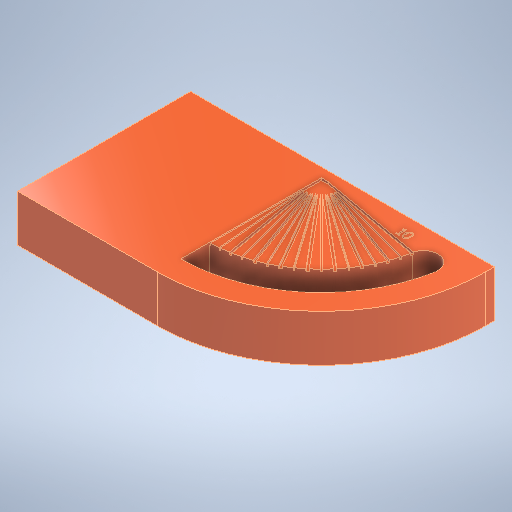
# Autodesk Inventor part: MainAnglePlate
Saved by Autodesk Inventor 2025.2 (Build 292293000, 293)
## iProperties
Created: 2025-03-13
Part Number: MainAnglePlate
Material: PET Plastic
Document SubType Name: Modeling
Designer: baolo
Density: 1.541 g/cm^3
Appearance: Smooth - Light Orange
Author: baolo
Autodesk Inventor part; units mm, degrees
ref_plane "YZ Plane" through (0, 0, 0) normal (1, 0, 0) x (0, 1, 0)
ref_plane "XZ Plane" through (0, 0, 0) normal (0, 1, 0) x (-1, 0, 0)
ref_plane "XY Plane" through (0, 0, 0) normal (0, 0, 1) x (1, 0, 0)
sketch "Sketch1" plane through (0, 0, 0) normal (0, 1, 0) x (-1, 0, 0)
  line L0 (35, 35) -> (-35, 35) construction
  line L1 (-35, 35) -> (-35, 0) construction
  line L2 (-35, 0) -> (35, 0)
  line L3 (35, 0) -> (35, 35) construction
  line L4 (35, 35) -> (-35, 0) construction
  line L5 (-35, 35) -> (35, 0) construction
  arc A0 (35, 0) -> (-35, 0) centre (0, 0) ccw
  line L6 (49, 0) -> (-49, 0) construction
  line L7 (0, -7) -> (0, 42) construction
  dimension "d0" = 70
  constraints: 12 end point, 2 midpoint, 2 parallel, 2 point on circle, 2 tangent, 1 centre point, 1 horizontal, 1 perpendicular, 1 point on line
  measures "d0" distance between parallel lines of L1 L3
extrude "Extrusion1" add sketch "Sketch1" along normal mid plane 10
sketch "Sketch3" plane through (0, 5, 0) normal (0, 1, 0) x (1, 0, 0)
  line L0 (35, 0) -> (-35, 0) construction
  arc A0 (-26.5898, -4.6885) -> (26.5898, -4.6885) centre (0, 0) ccw construction
  arc A1 (-29.5935, -5.2181) -> (29.5935, -5.2181) centre (0, 0) ccw
  arc A2 (-23.5861, -4.1589) -> (23.5861, -4.1589) centre (0, 0) ccw
  arc A3 (-23.5861, -4.1589) -> (-29.5935, -5.2181) centre (-26.5898, -4.6885) ccw
  arc A4 (29.5935, -5.2181) -> (23.5861, -4.1589) centre (26.5898, -4.6885) ccw
  arc A5 (-35, 0) -> (35, 0) centre (0, 0) ccw construction
  line L1 (-26.5898, -4.6885) -> (0, 0) construction
  line L2 (0, 0) -> (26.5898, -4.6885) construction
  dimension "d5" = 8
  dimension "d6" = 3.05
  dimension "d29" = 10
  constraints: 10 point on circle, 5 centre point, 4 end point, 4 tangent, 1 horizontal alignment, 1 midpoint
  measures "d5" radial gap between concentric circles of A5 A0
  measures "d6" radius of A3
  measures "d29" angle of L0 L2
extrude "Extrusion2" cut sketch "Sketch3" against normal through all
sketch "Sketch4" plane through (0, 5, 0) normal (0, 1, 0) x (1, 0, 0)
  line L0 (0.0434, 0.2462) -> (26.6321, -4.4421)
  line L1 (26.6321, -4.4421) -> (26.5453, -4.9345)
  line L2 (26.5453, -4.9345) -> (-0.0434, -0.2462)
  line L3 (-0.0434, -0.2462) -> (0.0434, 0.2462)
  arc A0 (-26.5018, -4.6885) -> (26.5886, -4.6885) centre (0.0434, 0.2462) ccw construction
  arc A1 (29.5935, -5.2181) -> (23.5861, -4.1589) centre (26.5898, -4.6885) ccw construction
  arc A2 (-23.5861, -4.1589) -> (-29.5935, -5.2181) centre (-26.5898, -4.6885) ccw construction
  line L4 (35, 0) -> (-35, 0) construction
  line L5 (0, 0) -> (26.5887, -4.6883) construction
  point P0 (0, 0)
  dimension "d10" = 27
  dimension "d11" = 0.5
  dimension "d23" = 10
  constraints: 11 end point, 3 midpoint, 3 perpendicular, 3 point on circle, 2 horizontal alignment, 1 centre point, 1 coincident, 1 parallel
  measures "d10" radius of A0
  measures "d11" distance between parallel lines of L2 L0
  measures "d23" angle of L4 L5
extrude "Extrusion3" cut sketch "Sketch4" against normal blind 0.5
pattern_circular "Circular Pattern1" count 19 over 180 about axis through (0, -10, 0) along (0, -1, 0) of "Extrusion3" skipped copies 18 19
sketch "Sketch5" plane through (0, 5, 0) normal (0, 1, 0) x (1, 0, 0)
  line L0 (35, 0) -> (1.4397, 0) construction
  arc A0 (-24.5564, -4.6885) -> (24.5564, -4.6885) centre (0, 0) ccw construction
  arc A1 (29.5935, -5.2181) -> (23.5861, -4.1589) centre (26.5898, -4.6885) ccw construction
  arc A2 (-23.5861, -4.1589) -> (-29.5935, -5.2181) centre (-26.5898, -4.6885) ccw construction
  line L1 (0.0324, 0.1207) -> (24.1805, -6.3497)
  line L2 (24.1805, -6.3497) -> (24.1158, -6.5912)
  line L3 (24.1158, -6.5912) -> (-0.0324, -0.1207)
  line L4 (-0.0324, -0.1207) -> (0.0324, 0.1207)
  line L5 (24.1481, -6.4705) -> (0, 0) construction
  dimension "d20" = 25
  dimension "d21" = 0.25
  dimension "d22" = 15
  constraints: 10 end point, 4 perpendicular, 3 point on circle, 2 coincident, 2 horizontal alignment, 2 midpoint, 1 centre point
  measures "d20" radius of A0
  measures "d21" distance between parallel lines of L3 L1
  measures "d22" angle of L0 L5
extrude "Extrusion4" cut sketch "Sketch5" against normal blind 0.5
pattern_circular "Circular Pattern2" count 19 over 180 about axis through (0, -10, 0) along (0, -1, 0) of "Extrusion4" skipped copies 17 18 19
sketch "Sketch6" plane through (0, 5, 0) normal (0, 1, 0) x (1, 0, 0)
  line L0 (17.9928, -0.4249) -> (37.6496, -0.4249) construction
  line L1 (37.6496, -0.4249) -> (37.6496, -4.495) construction
  line L2 (37.6496, -4.495) -> (17.9928, -4.495) construction
  line L3 (17.9928, -4.495) -> (17.9928, -0.4249) construction
  line L4 (18.8635, -2.3542) -> (18.6187, -2.3542)
  line L5 (18.6187, -2.3542) -> (18.3739, -2.3525)
  spline S0 degree 2 poles (18.3739, -2.3525) (18.2877, -2.3525) (18.2532, -2.3421) knots 0 0 0 1 1 1
  spline S1 degree 2 poles (18.2532, -2.3421) (18.1894, -2.3197) (18.1894, -2.2473) knots 0 0 0 1 1 1
  spline S2 degree 2 poles (18.1894, -2.2473) (18.1894, -2.1231) (18.3825, -2.1231) knots 0 0 0 1 1 1
  line L6 (18.3825, -2.1231) -> (18.4428, -2.1249)
  line L7 (18.4428, -2.1249) -> (18.4928, -2.1266)
  spline S3 degree 2 poles (18.4928, -2.1266) (18.4928, -2.068) (18.4721, -1.8352) (18.4721, -1.7766) knots 0 0 0 1 2 2 2
  spline S4 degree 2 poles (18.4721, -1.7766) (18.4721, -1.6197) (18.4997, -1.299) knots 0 0 0 1 1 1
  spline S5 degree 2 poles (18.4997, -1.299) (18.5273, -0.9852) (18.5256, -0.8214) knots 0 0 0 1 1 1
  spline S6 degree 2 poles (18.5256, -0.8214) (18.3601, -0.9507) (18.3152, -0.9507) knots 0 0 0 1 1 1
  spline S7 degree 2 poles (18.3152, -0.9507) (18.2652, -0.9507) (18.1928, -0.8766) (18.1928, -0.8283) knots 0 0 0 1 2 2 2
  spline S8 degree 2 poles (18.1928, -0.8283) (18.1928, -0.7697) (18.2997, -0.6869) knots 0 0 0 1 1 1
  spline S9 degree 2 poles (18.2997, -0.6869) (18.3652, -0.6387) (18.4877, -0.5352) knots 0 0 0 1 1 1
  spline S10 degree 2 poles (18.4877, -0.5352) (18.598, -0.4249) (18.6963, -0.4249) knots 0 0 0 1 1 1
  spline S11 degree 2 poles (18.6963, -0.4249) (18.779, -0.4249) (18.779, -0.5197) knots 0 0 0 1 1 1
  spline S12 degree 2 poles (18.779, -0.5197) (18.779, -0.549) (18.7635, -0.6611) (18.7635, -0.6904) knots 0 0 0 1 2 2 2
  spline S13 degree 2 poles (18.7635, -0.6904) (18.7635, -0.73) (18.7721, -0.8956) (18.7721, -0.9369) knots 0 0 0 1 2 2 2
  spline S14 degree 2 poles (18.7721, -0.9369) (18.7721, -1.0783) (18.7135, -1.6369) (18.7135, -1.7766) knots 0 0 0 1 2 2 2
  spline S15 degree 2 poles (18.7135, -1.7766) (18.7135, -1.849) (18.7325, -2.0542) (18.7342, -2.1197) knots 0 0 0 1 2 2 2
  line L8 (18.7342, -2.1197) -> (18.8635, -2.118)
  spline S16 degree 2 poles (18.8635, -2.118) (18.917, -2.118) (18.9842, -2.1852) (18.9842, -2.2352) knots 0 0 0 1 2 2 2
  spline S17 degree 2 poles (18.9842, -2.2352) (18.9842, -2.2869) (18.917, -2.3542) (18.8635, -2.3542) knots 0 0 0 1 2 2 2
  spline S18 degree 2 poles (19.8894, -2.4007) (19.5135, -2.4007) (19.3411, -2.0576) knots 0 0 0 1 1 1
  spline S19 degree 2 poles (19.3411, -2.0576) (19.2101, -1.7921) (19.2101, -1.368) knots 0 0 0 1 1 1
  spline S20 degree 2 poles (19.2101, -1.368) (19.2101, -1.0093) (19.3808, -0.7421) knots 0 0 0 1 1 1
  spline S21 degree 2 poles (19.3808, -0.7421) (19.5825, -0.43) (19.9273, -0.43) knots 0 0 0 1 1 1
  spline S22 degree 2 poles (19.9273, -0.43) (20.2532, -0.43) (20.4342, -0.7076) knots 0 0 0 1 1 1
  spline S23 degree 2 poles (20.4342, -0.7076) (20.5911, -0.9473) (20.5911, -1.2921) knots 0 0 0 1 1 1
  spline S24 degree 2 poles (20.5911, -1.2921) (20.5911, -1.8456) (20.2411, -2.4007) (19.8894, -2.4007) knots 0 0 0 1 2 2 2
  spline S25 degree 2 poles (19.9273, -0.668) (19.6963, -0.668) (19.5618, -0.9025) knots 0 0 0 1 1 1
  spline S26 degree 2 poles (19.5618, -0.9025) (19.4497, -1.0973) (19.4497, -1.3473) knots 0 0 0 1 1 1
  spline S27 degree 2 poles (19.4497, -1.3473) (19.4497, -1.7542) (19.6704, -2.1628) (19.8894, -2.1628) knots 0 0 0 1 2 2 2
  spline S28 degree 2 poles (19.8894, -2.1628) (20.1514, -2.1628) (20.2652, -1.8628) knots 0 0 0 1 1 1
  spline S29 degree 2 poles (20.2652, -1.8628) (20.3445, -1.6559) (20.3445, -1.3369) knots 0 0 0 1 1 1
  spline S30 degree 2 poles (20.3445, -1.3369) (20.3445, -1.0025) (20.1359, -0.668) (19.9273, -0.668) knots 0 0 0 1 2 2 2
  point P0 (0, 0)
  constraints: 2 other
emboss "Emboss1" sketch "Sketch6" operation cut depth 1 direction (0, -1, 0)
sketch "Sketch7" plane through (0, 5, 0) normal (0, 1, 0) x (1, 0, 0)
  line L0 (0, 0) -> (-69.9459, 0)
  line L1 (-69.9459, 0) -> (-69.9459, -63.8615)
  line L2 (-69.9459, -63.8615) -> (0, -63.8615)
  line L3 (0, -63.8615) -> (0, 0)
  constraints: 8 end point, 2 parallel, 1 horizontal, 1 perpendicular
extrude "Extrusion5" cut sketch "Sketch7" against normal through all
sketch "Sketch8" plane through (0, 0, 44.9993) normal (-1, 0, 0) x (0, 0, 1)
  line L0 (-44.9993, -5) -> (-44.9993, 4.5) construction
  line L1 (-9.9993, 5) -> (-9.9993, -5) construction
  line L2 (-44.9993, -5) -> (-44.9993, 5) projected
  line L3 (-44.9993, -5) -> (-9.9993, -5)
  line L4 (-9.9993, -5) -> (-9.9993, 5)
  line L5 (-9.9993, 5) -> (-44.9993, 5)
  line L6 (-44.9993, 5) -> (-44.9993, -5)
  point P0 (-44.9993, 5)
  constraints: 8 end point, 2 parallel, 1 horizontal, 1 perpendicular
extrude "Extrusion6" add sketch "Sketch8" along normal blind 30
sketch "Sketch10" plane through (0, -5, 0) normal (0, -1, 0) x (1, 0, 0)
  line L0 (5.7394, 2.8439) -> (-28.2134, 2.8439) construction
  line L1 (-28.2134, 2.8439) -> (-28.2134, 16.771) construction
  line L2 (-28.2134, 16.771) -> (5.7394, 16.771) construction
  line L3 (5.7394, 16.771) -> (5.7394, 2.8439) construction
  spline S0 degree 2 poles (3.3633, 4.9557) (3.3633, 5.183) (3.5362, 5.5312) (3.6794, 5.6448) knots 0 0 0 1 2 2 2
  spline S1 degree 2 poles (3.6794, 5.6448) (3.8523, 5.7782) (4.245, 5.8919) (4.5563, 5.8919) knots 0 0 0 1 2 2 2
  line L4 (4.5563, 5.8919) -> (5.4307, 5.8919)
  line L5 (5.4307, 5.8919) -> (5.4307, 2.8439)
  line L6 (5.4307, 2.8439) -> (4.623, 2.8439)
  spline S2 degree 2 poles (4.623, 2.8439) (4.2969, 2.8439) (3.9709, 2.8858) (3.8227, 2.9674) knots 0 0 0 1 2 2 2
  spline S3 degree 2 poles (3.8227, 2.9674) (3.6572, 3.0538) (3.5065, 3.3379) (3.5065, 3.5305) knots 0 0 0 1 2 2 2
  spline S4 degree 2 poles (3.5065, 3.5305) (3.5065, 3.7454) (3.7338, 4.0863) (3.9338, 4.1826) knots 0 0 0 1 2 2 2
  line L7 (3.9338, 4.1826) -> (3.9338, 4.1974)
  spline S5 degree 2 poles (3.9338, 4.1974) (3.6621, 4.2715) (3.3633, 4.6643) (3.3633, 4.9557) knots 0 0 0 1 2 2 2
  spline S6 degree 2 poles (3.7856, 4.973) (3.7856, 4.8001) (3.8844, 4.5778) (4.0326, 4.4988) knots 0 0 0 1 2 2 2
  spline S7 degree 2 poles (4.0326, 4.4988) (4.129, 4.4494) (4.3562, 4.4197) (4.5661, 4.4197) knots 0 0 0 1 2 2 2
  line L8 (4.5661, 4.4197) -> (5.0256, 4.4197)
  line L9 (5.0256, 4.4197) -> (5.0256, 5.546)
  line L10 (5.0256, 5.546) -> (4.6971, 5.546)
  spline S8 degree 2 poles (4.6971, 5.546) (4.4303, 5.546) (4.124, 5.4966) (4.0055, 5.4176) knots 0 0 0 1 2 2 2
  spline S9 degree 2 poles (4.0055, 5.4176) (3.8918, 5.3361) (3.7856, 5.1336) (3.7856, 4.973) knots 0 0 0 1 2 2 2
  spline S10 degree 2 poles (3.9289, 3.5873) (3.9289, 3.4786) (4.003, 3.3156) (4.0845, 3.2687) knots 0 0 0 1 2 2 2
  spline S11 degree 2 poles (4.0845, 3.2687) (4.1833, 3.2144) (4.4229, 3.1897) (4.6378, 3.1897) knots 0 0 0 1 2 2 2
  line L11 (4.6378, 3.1897) -> (5.0256, 3.1897)
  line L12 (5.0256, 3.1897) -> (5.0256, 4.0813)
  line L13 (5.0256, 4.0813) -> (4.5661, 4.0813)
  spline S12 degree 2 poles (4.5661, 4.0813) (4.376, 4.0813) (4.1956, 4.0418) (4.0993, 3.9801) knots 0 0 0 1 2 2 2
  spline S13 degree 2 poles (4.0993, 3.9801) (4.0055, 3.9208) (3.9289, 3.7306) (3.9289, 3.5873) knots 0 0 0 1 2 2 2
  spline S14 degree 2 poles (1.7158, 5.6498) (1.7627, 5.6844) (1.9208, 5.8079) (1.9949, 5.8449) knots 0 0 0 1 2 2 2
  spline S15 degree 2 poles (1.9949, 5.8449) (2.0961, 5.8993) (2.2863, 5.9561) (2.4592, 5.9561) knots 0 0 0 1 2 2 2
  spline S16 degree 2 poles (2.4592, 5.9561) (2.6, 5.9561) (2.8544, 5.8499) (2.9508, 5.7535) knots 0 0 0 1 2 2 2
  spline S17 degree 2 poles (2.9508, 5.7535) (3.0421, 5.6597) (3.1533, 5.383) (3.1533, 5.2299) knots 0 0 0 1 2 2 2
  spline S18 degree 2 poles (3.1533, 5.2299) (3.1533, 4.9928) (2.9532, 4.6568) (2.7359, 4.5605) knots 0 0 0 1 2 2 2
  spline S19 degree 2 poles (2.7359, 4.5605) (2.5432, 4.4716) (2.0196, 4.4049) (1.7158, 4.3876) knots 0 0 0 1 2 2 2
  line L14 (1.7158, 4.3876) -> (1.7158, 4.3135)
  spline S20 degree 2 poles (1.7158, 4.3135) (1.7158, 4.1801) (1.7973, 4.0146) (1.8714, 3.9677) knots 0 0 0 1 2 2 2
  spline S21 degree 2 poles (1.8714, 3.9677) (1.9455, 3.9208) (2.1579, 3.8911) (2.2715, 3.8911) knots 0 0 0 1 2 2 2
  spline S22 degree 2 poles (2.2715, 3.8911) (2.4049, 3.8911) (2.7655, 3.9702) (2.9458, 4.0467) knots 0 0 0 1 2 2 2
  line L15 (2.9458, 4.0467) -> (2.968, 4.0467)
  line L16 (2.968, 4.0467) -> (2.968, 3.654)
  spline S23 degree 2 poles (2.968, 3.654) (2.8618, 3.6244) (2.4642, 3.5503) (2.269, 3.5503) knots 0 0 0 1 2 2 2
  spline S24 degree 2 poles (2.269, 3.5503) (2.0319, 3.5503) (1.7083, 3.6244) (1.5799, 3.7207) knots 0 0 0 1 2 2 2
  spline S25 degree 2 poles (1.5799, 3.7207) (1.4539, 3.8146) (1.3304, 4.1134) (1.3304, 4.3283) knots 0 0 0 1 2 2 2
  line L17 (1.3304, 4.3283) -> (1.3304, 5.8919)
  line L18 (1.3304, 5.8919) -> (1.7158, 5.8919)
  line L19 (1.7158, 5.8919) -> (1.7158, 5.6498)
  line L20 (1.7158, 5.3287) -> (1.7158, 4.6939)
  spline S26 degree 2 poles (1.7158, 4.6939) (1.8541, 4.7062) (2.2715, 4.7482) (2.4024, 4.7878) knots 0 0 0 1 2 2 2
  spline S27 degree 2 poles (2.4024, 4.7878) (2.5556, 4.8347) (2.7556, 5.0298) (2.7556, 5.2027) knots 0 0 0 1 2 2 2
  spline S28 degree 2 poles (2.7556, 5.2027) (2.7556, 5.4003) (2.5333, 5.6004) (2.3209, 5.6004) knots 0 0 0 1 2 2 2
  spline S29 degree 2 poles (2.3209, 5.6004) (2.1406, 5.6004) (1.8442, 5.4448) (1.7158, 5.3287) knots 0 0 0 1 2 2 2
  spline S30 degree 2 poles (-1.0902, 4.7482) (-1.0902, 5.3262) (-0.5344, 5.9561) (-0.0701, 5.9561) knots 0 0 0 1 2 2 2
  spline S31 degree 2 poles (-0.0701, 5.9561) (0.4066, 5.9561) (0.9525, 5.3065) (0.9525, 4.7482) knots 0 0 0 1 2 2 2
  spline S32 degree 2 poles (0.9525, 4.7482) (0.9525, 4.1752) (0.3894, 3.5404) (-0.0701, 3.5404) knots 0 0 0 1 2 2 2
  spline S33 degree 2 poles (-0.0701, 3.5404) (-0.5344, 3.5404) (-1.0902, 4.1727) (-1.0902, 4.7482) knots 0 0 0 1 2 2 2
  spline S34 degree 2 poles (-0.6925, 4.7482) (-0.6925, 4.3036) (-0.3689, 3.8714) (-0.0701, 3.8714) knots 0 0 0 1 2 2 2
  spline S35 degree 2 poles (-0.0701, 3.8714) (0.2288, 3.8714) (0.5548, 4.3036) (0.5548, 4.7482) knots 0 0 0 1 2 2 2
  spline S36 degree 2 poles (0.5548, 4.7482) (0.5548, 5.1805) (0.2288, 5.6251) (-0.0701, 5.6251) knots 0 0 0 1 2 2 2
  spline S37 degree 2 poles (-0.0701, 5.6251) (-0.3665, 5.6251) (-0.6925, 5.1879) (-0.6925, 4.7482) knots 0 0 0 1 2 2 2
  line L21 (-5.0052, 5.8919) -> (-4.5507, 5.8919)
  line L22 (-4.5507, 5.8919) -> (-3.2021, 3.2638)
  line L23 (-3.2021, 3.2638) -> (-3.2021, 5.8919)
  line L24 (-3.2021, 5.8919) -> (-2.8241, 5.8919)
  line L25 (-2.8241, 5.8919) -> (-2.8241, 2.8439)
  line L26 (-2.8241, 2.8439) -> (-3.3997, 2.8439)
  line L27 (-3.3997, 2.8439) -> (-4.6273, 5.2571)
  line L28 (-4.6273, 5.2571) -> (-4.6273, 2.8439)
  line L29 (-4.6273, 2.8439) -> (-5.0052, 2.8439)
  line L30 (-5.0052, 2.8439) -> (-5.0052, 5.8919)
  line L31 (-6.1908, 5.8919) -> (-5.7017, 5.8919)
  line L32 (-5.7017, 5.8919) -> (-5.7017, 5.3089)
  line L33 (-5.7017, 5.3089) -> (-6.1908, 5.3089)
  line L34 (-6.1908, 5.3089) -> (-6.1908, 5.8919)
  line L35 (4.287, 11.7526) -> (4.7563, 11.7526)
  spline S38 degree 2 poles (4.7563, 11.7526) (5.112, 11.3302) (5.5196, 10.3842) (5.5196, 9.7395) knots 0 0 0 1 2 2 2
  spline S39 degree 2 poles (5.5196, 9.7395) (5.5196, 9.1097) (5.117, 8.1488) (4.7563, 7.7265) knots 0 0 0 1 2 2 2
  line L36 (4.7563, 7.7265) -> (4.287, 7.7265)
  line L37 (4.287, 7.7265) -> (4.287, 7.7462)
  spline S40 degree 2 poles (4.287, 7.7462) (4.4525, 7.8969) (4.7539, 8.2871) (4.8823, 8.5465) knots 0 0 0 1 2 2 2
  spline S41 degree 2 poles (4.8823, 8.5465) (5.0058, 8.7984) (5.159, 9.4036) (5.159, 9.7395) knots 0 0 0 1 2 2 2
  spline S42 degree 2 poles (5.159, 9.7395) (5.159, 10.0903) (5.0108, 10.6707) (4.8823, 10.9325) knots 0 0 0 1 2 2 2
  spline S43 degree 2 poles (4.8823, 10.9325) (4.7588, 11.1845) (4.4451, 11.592) (4.287, 11.7328) knots 0 0 0 1 2 2 2
  line L38 (4.287, 11.7328) -> (4.287, 11.7526)
  line L39 (3.8251, 10.9103) -> (3.8251, 7.8623)
  line L40 (3.8251, 7.8623) -> (1.9183, 7.8623)
  line L41 (1.9183, 7.8623) -> (1.9183, 8.2229)
  line L42 (1.9183, 8.2229) -> (3.4201, 8.2229)
  line L43 (3.4201, 8.2229) -> (3.4201, 9.0578)
  line L44 (3.4201, 9.0578) -> (2.0196, 9.0578)
  line L45 (2.0196, 9.0578) -> (2.0196, 9.4184)
  line L46 (2.0196, 9.4184) -> (3.4201, 9.4184)
  line L47 (3.4201, 9.4184) -> (3.4201, 10.5497)
  line L48 (3.4201, 10.5497) -> (1.9183, 10.5497)
  line L49 (1.9183, 10.5497) -> (1.9183, 10.9103)
  line L50 (1.9183, 10.9103) -> (3.8251, 10.9103)
  line L51 (-0.3195, 10.9103) -> (1.5601, 10.9103)
  line L52 (1.5601, 10.9103) -> (1.5601, 10.478)
  spline S44 degree 2 poles (1.5601, 10.478) (1.3576, 10.2879) (0.997, 9.9346) (0.8241, 9.7445) knots 0 0 0 1 2 2 2
  spline S45 degree 2 poles (0.8241, 9.7445) (0.4758, 9.3616) (0.2214, 8.9022) (0.2214, 8.6576) knots 0 0 0 1 2 2 2
  spline S46 degree 2 poles (0.2214, 8.6576) (0.2214, 8.5292) (0.3004, 8.3365) (0.3721, 8.2748) knots 0 0 0 1 2 2 2
  spline S47 degree 2 poles (0.3721, 8.2748) (0.4437, 8.213) (0.6314, 8.1513) (0.745, 8.1513) knots 0 0 0 1 2 2 2
  spline S48 degree 2 poles (0.745, 8.1513) (0.8537, 8.1513) (1.076, 8.2056) (1.1773, 8.2476) knots 0 0 0 1 2 2 2
  spline S49 degree 2 poles (1.1773, 8.2476) (1.2637, 8.2822) (1.4243, 8.381) (1.4737, 8.4156) knots 0 0 0 1 2 2 2
  line L53 (1.4737, 8.4156) -> (1.4959, 8.4156)
  line L54 (1.4959, 8.4156) -> (1.4959, 7.9809)
  spline S50 degree 2 poles (1.4959, 7.9809) (1.3699, 7.9191) (0.9179, 7.7981) (0.7154, 7.7981) knots 0 0 0 1 2 2 2
  spline S51 degree 2 poles (0.7154, 7.7981) (0.2881, 7.7981) (-0.1936, 8.2501) (-0.1936, 8.6354) knots 0 0 0 1 2 2 2
  spline S52 degree 2 poles (-0.1936, 8.6354) (-0.1936, 8.8157) (-0.1096, 9.1171) (-0.0355, 9.2455) knots 0 0 0 1 2 2 2
  spline S53 degree 2 poles (-0.0355, 9.2455) (0.0386, 9.3789) (0.2535, 9.6407) (0.3721, 9.7667) knots 0 0 0 1 2 2 2
  spline S54 degree 2 poles (0.3721, 9.7667) (0.5647, 9.9766) (1.0365, 10.4262) (1.1773, 10.5571) knots 0 0 0 1 2 2 2
  line L55 (1.1773, 10.5571) -> (-0.3195, 10.5571)
  line L56 (-0.3195, 10.5571) -> (-0.3195, 10.9103)
  line L57 (-1.8435, 9.7617) -> (-0.69, 9.7617)
  line L58 (-0.69, 9.7617) -> (-0.69, 9.3912)
  line L59 (-0.69, 9.3912) -> (-1.8435, 9.3912)
  line L60 (-1.8435, 9.3912) -> (-1.8435, 9.7617)
  line L61 (-3.9752, 10.9103) -> (-2.4882, 10.9103)
  line L62 (-2.4882, 10.9103) -> (-2.4882, 10.5991)
  line L63 (-2.4882, 10.5991) -> (-3.0415, 10.5991)
  line L64 (-3.0415, 10.5991) -> (-3.0415, 8.5564)
  line L65 (-3.0415, 8.5564) -> (-2.4882, 8.5564)
  line L66 (-2.4882, 8.5564) -> (-2.4882, 8.2773)
  spline S55 degree 2 poles (-2.4882, 8.2773) (-2.8019, 8.2773) (-3.0983, 8.0994) (-3.1181, 7.8524) knots 0 0 0 1 2 2 2
  line L67 (-3.1181, 7.8524) -> (-3.4342, 7.8524)
  line L68 (-3.4342, 7.8524) -> (-3.4342, 10.5991)
  line L69 (-3.4342, 10.5991) -> (-3.9752, 10.5991)
  line L70 (-3.9752, 10.5991) -> (-3.9752, 10.9103)
  spline S56 degree 2 poles (-5.3584, 8.1513) (-5.2472, 8.1513) (-5.0274, 8.2056) (-4.9212, 8.2476) knots 0 0 0 1 2 2 2
  spline S57 degree 2 poles (-4.9212, 8.2476) (-4.8224, 8.2896) (-4.6767, 8.3785) (-4.6198, 8.4181) knots 0 0 0 1 2 2 2
  line L71 (-4.6198, 8.4181) -> (-4.5951, 8.4181)
  line L72 (-4.5951, 8.4181) -> (-4.5951, 7.9858)
  spline S58 degree 2 poles (-4.5951, 7.9858) (-4.7285, 7.9142) (-5.1855, 7.7981) (-5.3905, 7.7981) knots 0 0 0 1 2 2 2
  spline S59 degree 2 poles (-5.3905, 7.7981) (-5.598, 7.7981) (-5.9067, 7.8821) (-6.0327, 7.971) knots 0 0 0 1 2 2 2
  spline S60 degree 2 poles (-6.0327, 7.971) (-6.1661, 8.0673) (-6.3044, 8.3464) (-6.3044, 8.5341) knots 0 0 0 1 2 2 2
  spline S61 degree 2 poles (-6.3044, 8.5341) (-6.3044, 8.7861) (-5.9734, 9.1665) (-5.7412, 9.2159) knots 0 0 0 1 2 2 2
  line L73 (-5.7412, 9.2159) -> (-5.7412, 9.2455)
  spline S62 degree 2 poles (-5.7412, 9.2455) (-5.8376, 9.2653) (-6.0574, 9.3542) (-6.1513, 9.4431) knots 0 0 0 1 2 2 2
  spline S63 degree 2 poles (-6.1513, 9.4431) (-6.2451, 9.5296) (-6.3637, 9.8062) (-6.3637, 10.0063) knots 0 0 0 1 2 2 2
  spline S64 degree 2 poles (-6.3637, 10.0063) (-6.3637, 10.2113) (-6.2229, 10.5596) (-6.0944, 10.6929) knots 0 0 0 1 2 2 2
  spline S65 degree 2 poles (-6.0944, 10.6929) (-5.9611, 10.8313) (-5.5831, 10.9745) (-5.3436, 10.9745) knots 0 0 0 1 2 2 2
  spline S66 degree 2 poles (-5.3436, 10.9745) (-5.1138, 10.9745) (-4.6643, 10.8634) (-4.5112, 10.7868) knots 0 0 0 1 2 2 2
  line L74 (-4.5112, 10.7868) -> (-4.5112, 10.3545)
  line L75 (-4.5112, 10.3545) -> (-4.5408, 10.3545)
  spline S67 degree 2 poles (-4.5408, 10.3545) (-4.6692, 10.4484) (-5.104, 10.6213) (-5.3189, 10.6213) knots 0 0 0 1 2 2 2
  spline S68 degree 2 poles (-5.3189, 10.6213) (-5.4448, 10.6213) (-5.6968, 10.5423) (-5.7807, 10.4509) knots 0 0 0 1 2 2 2
  spline S69 degree 2 poles (-5.7807, 10.4509) (-5.8623, 10.3595) (-5.9487, 10.1421) (-5.9487, 9.9766) knots 0 0 0 1 2 2 2
  spline S70 degree 2 poles (-5.9487, 9.9766) (-5.9487, 9.8111) (-5.8524, 9.5963) (-5.7659, 9.5345) knots 0 0 0 1 2 2 2
  spline S71 degree 2 poles (-5.7659, 9.5345) (-5.6795, 9.4728) (-5.4448, 9.4258) (-5.3065, 9.4258) knots 0 0 0 1 2 2 2
  line L76 (-5.3065, 9.4258) -> (-5.1336, 9.4258)
  line L77 (-5.1336, 9.4258) -> (-5.1336, 9.0874)
  line L78 (-5.1336, 9.0874) -> (-5.2695, 9.0874)
  spline S72 degree 2 poles (-5.2695, 9.0874) (-5.5436, 9.0874) (-5.8894, 8.8256) (-5.8894, 8.5761) knots 0 0 0 1 2 2 2
  spline S73 degree 2 poles (-5.8894, 8.5761) (-5.8894, 8.46) (-5.8005, 8.2946) (-5.7289, 8.2452) knots 0 0 0 1 2 2 2
  spline S74 degree 2 poles (-5.7289, 8.2452) (-5.6523, 8.1933) (-5.4646, 8.1513) (-5.3584, 8.1513) knots 0 0 0 1 2 2 2
  line L79 (-8.93, 10.9103) -> (-8.93, 8.2229)
  line L80 (-8.93, 8.2229) -> (-7.9074, 8.2229)
  line L81 (-7.9074, 8.2229) -> (-7.9074, 7.8623)
  line L82 (-7.9074, 7.8623) -> (-10.3577, 7.8623)
  line L83 (-10.3577, 7.8623) -> (-10.3577, 8.2229)
  line L84 (-10.3577, 8.2229) -> (-9.3351, 8.2229)
  line L85 (-9.3351, 8.2229) -> (-9.3351, 10.9103)
  line L86 (-9.3351, 10.9103) -> (-8.93, 10.9103)
  line L87 (-11.8496, 9.0356) -> (-11.8298, 9.0356)
  spline S75 degree 2 poles (-11.8298, 9.0356) (-11.7854, 9.0232) (-11.689, 9.0183) (-11.6223, 9.0183) knots 0 0 0 1 2 2 2
  spline S76 degree 2 poles (-11.6223, 9.0183) (-11.4667, 9.0183) (-11.1604, 9.1541) (-11.0221, 9.2875) knots 0 0 0 1 2 2 2
  line L88 (-11.0221, 9.2875) -> (-11.0221, 10.9103)
  line L89 (-11.0221, 10.9103) -> (-10.6368, 10.9103)
  line L90 (-10.6368, 10.9103) -> (-10.6368, 8.6231)
  line L91 (-10.6368, 8.6231) -> (-11.0221, 8.6231)
  line L92 (-11.0221, 8.6231) -> (-11.0221, 8.9639)
  spline S77 degree 2 poles (-11.0221, 8.9639) (-11.2321, 8.7762) (-11.5458, 8.6231) (-11.694, 8.6231) knots 0 0 0 1 2 2 2
  spline S78 degree 2 poles (-11.694, 8.6231) (-11.7532, 8.6231) (-11.8125, 8.628) (-11.8496, 8.6354) knots 0 0 0 1 2 2 2
  line L93 (-11.8496, 8.6354) -> (-11.8496, 9.0356)
  spline S79 degree 2 poles (-13.1414, 10.9622) (-12.5931, 10.9622) (-11.9904, 10.3471) (-11.9904, 9.779) knots 0 0 0 1 2 2 2
  spline S80 degree 2 poles (-11.9904, 9.779) (-11.9904, 9.2208) (-12.5758, 8.5588) (-13.0475, 8.5588) knots 0 0 0 1 2 2 2
  spline S81 degree 2 poles (-13.0475, 8.5588) (-13.26, 8.5588) (-13.5885, 8.6823) (-13.7095, 8.8133) knots 0 0 0 1 2 2 2
  spline S82 degree 2 poles (-13.7095, 8.8133) (-13.833, 8.9442) (-13.9639, 9.3221) (-13.9639, 9.5963) knots 0 0 0 1 2 2 2
  line L94 (-13.9639, 9.5963) -> (-13.9639, 9.8062)
  line L95 (-13.9639, 9.8062) -> (-12.3806, 9.8062)
  spline S83 degree 2 poles (-12.3806, 9.8062) (-12.3806, 10.2039) (-12.7808, 10.6263) (-13.1365, 10.6263) knots 0 0 0 1 2 2 2
  spline S84 degree 2 poles (-13.1365, 10.6263) (-13.2624, 10.6263) (-13.507, 10.5694) (-13.6058, 10.525) knots 0 0 0 1 2 2 2
  spline S85 degree 2 poles (-13.6058, 10.525) (-13.7095, 10.4756) (-13.8528, 10.3891) (-13.8997, 10.3496) knots 0 0 0 1 2 2 2
  line L96 (-13.8997, 10.3496) -> (-13.9219, 10.3496)
  line L97 (-13.9219, 10.3496) -> (-13.9219, 10.7695)
  spline S86 degree 2 poles (-13.9219, 10.7695) (-13.8552, 10.7967) (-13.6527, 10.8757) (-13.5736, 10.898) knots 0 0 0 1 2 2 2
  spline S87 degree 2 poles (-13.5736, 10.898) (-13.4625, 10.9301) (-13.2797, 10.9622) (-13.1414, 10.9622) knots 0 0 0 1 2 2 2
  spline S88 degree 2 poles (-13.5885, 9.5123) (-13.5835, 9.3567) (-13.5193, 9.1294) (-13.4576, 9.0529) knots 0 0 0 1 2 2 2
  spline S89 degree 2 poles (-13.4576, 9.0529) (-13.3909, 8.9664) (-13.1809, 8.875) (-13.0253, 8.875) knots 0 0 0 1 2 2 2
  spline S90 degree 2 poles (-13.0253, 8.875) (-12.8722, 8.875) (-12.6573, 8.9664) (-12.5684, 9.0553) knots 0 0 0 1 2 2 2
  spline S91 degree 2 poles (-12.5684, 9.0553) (-12.4819, 9.1467) (-12.393, 9.3665) (-12.3806, 9.5123) knots 0 0 0 1 2 2 2
  line L98 (-12.3806, 9.5123) -> (-13.5885, 9.5123)
  spline S92 degree 2 poles (-16.2709, 9.7296) (-16.2709, 10.2903) (-15.7275, 10.9745) (-15.3175, 10.9745) knots 0 0 0 1 2 2 2
  spline S93 degree 2 poles (-15.3175, 10.9745) (-15.1322, 10.9745) (-14.8679, 10.8831) (-14.7395, 10.8041) knots 0 0 0 1 2 2 2
  line L99 (-14.7395, 10.8041) -> (-14.7148, 10.9103)
  line L100 (-14.7148, 10.9103) -> (-14.3542, 10.9103)
  line L101 (-14.3542, 10.9103) -> (-14.3542, 7.7265)
  line L102 (-14.3542, 7.7265) -> (-14.7395, 7.7265)
  line L103 (-14.7395, 7.7265) -> (-14.7395, 8.8627)
  spline S94 degree 2 poles (-14.7395, 8.8627) (-14.8852, 8.7317) (-15.2236, 8.5588) (-15.4385, 8.5588) knots 0 0 0 1 2 2 2
  spline S95 degree 2 poles (-15.4385, 8.5588) (-15.8263, 8.5588) (-16.2709, 9.1788) (-16.2709, 9.7296) knots 0 0 0 1 2 2 2
  spline S96 degree 2 poles (-15.8732, 9.7593) (-15.8732, 9.3493) (-15.6238, 8.9244) (-15.3471, 8.9244) knots 0 0 0 1 2 2 2
  spline S97 degree 2 poles (-15.3471, 8.9244) (-15.1915, 8.9244) (-14.8704, 9.0726) (-14.7395, 9.1862) knots 0 0 0 1 2 2 2
  line L104 (-14.7395, 9.1862) -> (-14.7395, 10.4978)
  spline S98 degree 2 poles (-14.7395, 10.4978) (-14.8852, 10.5694) (-15.11, 10.6287) (-15.2434, 10.6287) knots 0 0 0 1 2 2 2
  spline S99 degree 2 poles (-15.2434, 10.6287) (-15.5373, 10.6287) (-15.8732, 10.2113) (-15.8732, 9.7593) knots 0 0 0 1 2 2 2
  line L105 (-18.4495, 10.9103) -> (-18.0641, 10.9103)
  line L106 (-18.0641, 10.9103) -> (-18.0641, 10.6584)
  spline S100 degree 2 poles (-18.0641, 10.6584) (-17.8863, 10.814) (-17.5677, 10.9745) (-17.3701, 10.9745) knots 0 0 0 1 2 2 2
  spline S101 degree 2 poles (-17.3701, 10.9745) (-17.2219, 10.9745) (-16.9576, 10.8757) (-16.8612, 10.7695) knots 0 0 0 1 2 2 2
  spline S102 degree 2 poles (-16.8612, 10.7695) (-16.7624, 10.6633) (-16.6538, 10.3397) (-16.6538, 10.1075) knots 0 0 0 1 2 2 2
  line L107 (-16.6538, 10.1075) -> (-16.6538, 8.6231)
  line L108 (-16.6538, 8.6231) -> (-17.0391, 8.6231)
  line L109 (-17.0391, 8.6231) -> (-17.0391, 9.9272)
  spline S103 degree 2 poles (-17.0391, 9.9272) (-17.0391, 10.11) (-17.0663, 10.3496) (-17.1132, 10.4385) knots 0 0 0 1 2 2 2
  spline S104 degree 2 poles (-17.1132, 10.4385) (-17.1601, 10.5275) (-17.3207, 10.609) (-17.4713, 10.609) knots 0 0 0 1 2 2 2
  spline S105 degree 2 poles (-17.4713, 10.609) (-17.6121, 10.609) (-17.9308, 10.4484) (-18.0641, 10.3323) knots 0 0 0 1 2 2 2
  line L110 (-18.0641, 10.3323) -> (-18.0641, 8.6231)
  line L111 (-18.0641, 8.6231) -> (-18.4495, 8.6231)
  line L112 (-18.4495, 8.6231) -> (-18.4495, 10.9103)
  spline S106 degree 2 poles (-19.9167, 10.9622) (-19.6795, 10.9622) (-19.2868, 10.8164) (-19.146, 10.6682) knots 0 0 0 1 2 2 2
  spline S107 degree 2 poles (-19.146, 10.6682) (-19.0052, 10.5225) (-18.8496, 10.073) (-18.8496, 9.7716) knots 0 0 0 1 2 2 2
  spline S108 degree 2 poles (-18.8496, 9.7716) (-18.8496, 9.4703) (-19.0102, 9.0306) (-19.146, 8.8824) knots 0 0 0 1 2 2 2
  spline S109 degree 2 poles (-19.146, 8.8824) (-19.2819, 8.7317) (-19.6845, 8.5712) (-19.9167, 8.5712) knots 0 0 0 1 2 2 2
  spline S110 degree 2 poles (-19.9167, 8.5712) (-20.1044, 8.5712) (-20.4551, 8.6774) (-20.591, 8.7466) knots 0 0 0 1 2 2 2
  line L113 (-20.591, 8.7466) -> (-20.591, 9.1788)
  line L114 (-20.591, 9.1788) -> (-20.5687, 9.1788)
  spline S111 degree 2 poles (-20.5687, 9.1788) (-20.5267, 9.1442) (-20.3983, 9.0553) (-20.3069, 9.0084) knots 0 0 0 1 2 2 2
  spline S112 degree 2 poles (-20.3069, 9.0084) (-20.2254, 8.9689) (-20.008, 8.9071) (-19.9092, 8.9071) knots 0 0 0 1 2 2 2
  spline S113 degree 2 poles (-19.9092, 8.9071) (-19.6104, 8.9071) (-19.2473, 9.3591) (-19.2473, 9.7716) knots 0 0 0 1 2 2 2
  spline S114 degree 2 poles (-19.2473, 9.7716) (-19.2473, 10.1742) (-19.598, 10.6263) (-19.9092, 10.6263) knots 0 0 0 1 2 2 2
  spline S115 degree 2 poles (-19.9092, 10.6263) (-20.097, 10.6263) (-20.4378, 10.4706) (-20.5687, 10.3496) knots 0 0 0 1 2 2 2
  line L115 (-20.5687, 10.3496) -> (-20.591, 10.3496)
  line L116 (-20.591, 10.3496) -> (-20.591, 10.7819)
  spline S116 degree 2 poles (-20.591, 10.7819) (-20.5342, 10.809) (-20.3613, 10.8856) (-20.2921, 10.9029) knots 0 0 0 1 2 2 2
  spline S117 degree 2 poles (-20.2921, 10.9029) (-20.1933, 10.9325) (-20.0377, 10.9622) (-19.9167, 10.9622) knots 0 0 0 1 2 2 2
  line L117 (-22.7374, 10.9103) -> (-22.3521, 10.9103)
  line L118 (-22.3521, 10.9103) -> (-22.3521, 9.6061)
  spline S118 degree 2 poles (-22.3521, 9.6061) (-22.3521, 9.4481) (-22.3224, 9.1764) (-22.278, 9.0948) knots 0 0 0 1 2 2 2
  spline S119 degree 2 poles (-22.278, 9.0948) (-22.2311, 9.0084) (-22.0631, 8.9244) (-21.9198, 8.9244) knots 0 0 0 1 2 2 2
  spline S120 degree 2 poles (-21.9198, 8.9244) (-21.7766, 8.9244) (-21.4728, 9.0776) (-21.327, 9.2011) knots 0 0 0 1 2 2 2
  line L119 (-21.327, 9.2011) -> (-21.327, 10.9103)
  line L120 (-21.327, 10.9103) -> (-20.9417, 10.9103)
  line L121 (-20.9417, 10.9103) -> (-20.9417, 7.7265)
  line L122 (-20.9417, 7.7265) -> (-21.327, 7.7265)
  line L123 (-21.327, 7.7265) -> (-21.327, 8.8775)
  spline S121 degree 2 poles (-21.327, 8.8775) (-21.4999, 8.7219) (-21.8334, 8.5588) (-22.0211, 8.5588) knots 0 0 0 1 2 2 2
  spline S122 degree 2 poles (-22.0211, 8.5588) (-22.357, 8.5588) (-22.7374, 9.0035) (-22.7374, 9.4258) knots 0 0 0 1 2 2 2
  line L124 (-22.7374, 9.4258) -> (-22.7374, 10.9103)
  spline S123 degree 2 poles (-24.2713, 10.9622) (-23.7229, 10.9622) (-23.1203, 10.3471) (-23.1203, 9.779) knots 0 0 0 1 2 2 2
  spline S124 degree 2 poles (-23.1203, 9.779) (-23.1203, 9.2208) (-23.7057, 8.5588) (-24.1774, 8.5588) knots 0 0 0 1 2 2 2
  spline S125 degree 2 poles (-24.1774, 8.5588) (-24.3899, 8.5588) (-24.7184, 8.6823) (-24.8394, 8.8133) knots 0 0 0 1 2 2 2
  spline S126 degree 2 poles (-24.8394, 8.8133) (-24.9629, 8.9442) (-25.0938, 9.3221) (-25.0938, 9.5963) knots 0 0 0 1 2 2 2
  line L125 (-25.0938, 9.5963) -> (-25.0938, 9.8062)
  line L126 (-25.0938, 9.8062) -> (-23.5105, 9.8062)
  spline S127 degree 2 poles (-23.5105, 9.8062) (-23.5105, 10.2039) (-23.9107, 10.6263) (-24.2663, 10.6263) knots 0 0 0 1 2 2 2
  spline S128 degree 2 poles (-24.2663, 10.6263) (-24.3923, 10.6263) (-24.6369, 10.5694) (-24.7357, 10.525) knots 0 0 0 1 2 2 2
  spline S129 degree 2 poles (-24.7357, 10.525) (-24.8394, 10.4756) (-24.9827, 10.3891) (-25.0296, 10.3496) knots 0 0 0 1 2 2 2
  line L127 (-25.0296, 10.3496) -> (-25.0518, 10.3496)
  line L128 (-25.0518, 10.3496) -> (-25.0518, 10.7695)
  spline S130 degree 2 poles (-25.0518, 10.7695) (-24.9851, 10.7967) (-24.7826, 10.8757) (-24.7035, 10.898) knots 0 0 0 1 2 2 2
  spline S131 degree 2 poles (-24.7035, 10.898) (-24.5924, 10.9301) (-24.4096, 10.9622) (-24.2713, 10.9622) knots 0 0 0 1 2 2 2
  spline S132 degree 2 poles (-24.7184, 9.5123) (-24.7134, 9.3567) (-24.6492, 9.1294) (-24.5875, 9.0529) knots 0 0 0 1 2 2 2
  spline S133 degree 2 poles (-24.5875, 9.0529) (-24.5208, 8.9664) (-24.3108, 8.875) (-24.1552, 8.875) knots 0 0 0 1 2 2 2
  spline S134 degree 2 poles (-24.1552, 8.875) (-24.0021, 8.875) (-23.7872, 8.9664) (-23.6982, 9.0553) knots 0 0 0 1 2 2 2
  spline S135 degree 2 poles (-23.6982, 9.0553) (-23.6118, 9.1467) (-23.5229, 9.3665) (-23.5105, 9.5123) knots 0 0 0 1 2 2 2
  line L129 (-23.5105, 9.5123) -> (-24.7184, 9.5123)
  spline S136 degree 2 poles (-26.1757, 10.9548) (-25.862, 10.9548) (-25.5088, 10.5966) (-25.5088, 10.2088) knots 0 0 0 1 2 2 2
  line L130 (-25.5088, 10.2088) -> (-25.5088, 8.9417)
  line L131 (-25.5088, 8.9417) -> (-25.2494, 8.9417)
  line L132 (-25.2494, 8.9417) -> (-25.2494, 8.6231)
  line L133 (-25.2494, 8.6231) -> (-25.5088, 8.6231)
  line L134 (-25.5088, 8.6231) -> (-25.5088, 7.966)
  line L135 (-25.5088, 7.966) -> (-25.8941, 7.966)
  line L136 (-25.8941, 7.966) -> (-25.8941, 8.6231)
  line L137 (-25.8941, 8.6231) -> (-26.603, 8.6231)
  line L138 (-26.603, 8.6231) -> (-26.603, 8.9417)
  line L139 (-26.603, 8.9417) -> (-25.8941, 8.9417)
  line L140 (-25.8941, 8.9417) -> (-25.8941, 10.031)
  spline S137 degree 2 poles (-25.8941, 10.031) (-25.8941, 10.2039) (-25.9064, 10.3941) (-25.9484, 10.4756) knots 0 0 0 1 2 2 2
  spline S138 degree 2 poles (-25.9484, 10.4756) (-25.983, 10.5472) (-26.1386, 10.6188) (-26.272, 10.6188) knots 0 0 0 1 2 2 2
  spline S139 degree 2 poles (-26.272, 10.6188) (-26.3659, 10.6188) (-26.5412, 10.562) (-26.5808, 10.5447) knots 0 0 0 1 2 2 2
  line L141 (-26.5808, 10.5447) -> (-26.603, 10.5447)
  line L142 (-26.603, 10.5447) -> (-26.603, 10.8905)
  spline S140 degree 2 poles (-26.603, 10.8905) (-26.4943, 10.9202) (-26.272, 10.9548) (-26.1757, 10.9548) knots 0 0 0 1 2 2 2
  spline S141 degree 2 poles (-27.9936, 9.7395) (-27.9936, 10.3718) (-27.5885, 11.3302) (-27.2304, 11.7526) knots 0 0 0 1 2 2 2
  line L143 (-27.2304, 11.7526) -> (-26.7611, 11.7526)
  line L144 (-26.7611, 11.7526) -> (-26.7611, 11.7328)
  spline S142 degree 2 poles (-26.7611, 11.7328) (-26.9191, 11.592) (-27.2378, 11.1795) (-27.3563, 10.9325) knots 0 0 0 1 2 2 2
  spline S143 degree 2 poles (-27.3563, 10.9325) (-27.4848, 10.6682) (-27.633, 10.0804) (-27.633, 9.7395) knots 0 0 0 1 2 2 2
  spline S144 degree 2 poles (-27.633, 9.7395) (-27.633, 9.4011) (-27.4823, 8.8009) (-27.3563, 8.5465) knots 0 0 0 1 2 2 2
  spline S145 degree 2 poles (-27.3563, 8.5465) (-27.2328, 8.2921) (-26.9167, 7.887) (-26.7611, 7.7462) knots 0 0 0 1 2 2 2
  line L145 (-26.7611, 7.7462) -> (-26.7611, 7.7265)
  line L146 (-26.7611, 7.7265) -> (-27.2304, 7.7265)
  spline S146 degree 2 poles (-27.2304, 7.7265) (-27.5861, 8.1488) (-27.9936, 9.1023) (-27.9936, 9.7395) knots 0 0 0 1 2 2 2
  line L147 (4.287, 16.771) -> (4.7563, 16.771)
  spline S147 degree 2 poles (4.7563, 16.771) (5.112, 16.3487) (5.5196, 15.4026) (5.5196, 14.758) knots 0 0 0 1 2 2 2
  spline S148 degree 2 poles (5.5196, 14.758) (5.5196, 14.1281) (5.117, 13.1673) (4.7563, 12.7449) knots 0 0 0 1 2 2 2
  line L148 (4.7563, 12.7449) -> (4.287, 12.7449)
  line L149 (4.287, 12.7449) -> (4.287, 12.7647)
  spline S149 degree 2 poles (4.287, 12.7647) (4.4525, 12.9153) (4.7539, 13.3056) (4.8823, 13.5649) knots 0 0 0 1 2 2 2
  spline S150 degree 2 poles (4.8823, 13.5649) (5.0058, 13.8169) (5.159, 14.422) (5.159, 14.758) knots 0 0 0 1 2 2 2
  spline S151 degree 2 poles (5.159, 14.758) (5.159, 15.1087) (5.0108, 15.6892) (4.8823, 15.951) knots 0 0 0 1 2 2 2
  spline S152 degree 2 poles (4.8823, 15.951) (4.7588, 16.2029) (4.4451, 16.6105) (4.287, 16.7513) knots 0 0 0 1 2 2 2
  line L150 (4.287, 16.7513) -> (4.287, 16.771)
  line L151 (3.8251, 15.9288) -> (3.8251, 12.8808)
  line L152 (3.8251, 12.8808) -> (1.9183, 12.8808)
  line L153 (1.9183, 12.8808) -> (1.9183, 13.2414)
  line L154 (1.9183, 13.2414) -> (3.4201, 13.2414)
  line L155 (3.4201, 13.2414) -> (3.4201, 14.0762)
  line L156 (3.4201, 14.0762) -> (2.0196, 14.0762)
  line L157 (2.0196, 14.0762) -> (2.0196, 14.4369)
  line L158 (2.0196, 14.4369) -> (3.4201, 14.4369)
  line L159 (3.4201, 14.4369) -> (3.4201, 15.5681)
  line L160 (3.4201, 15.5681) -> (1.9183, 15.5681)
  line L161 (1.9183, 15.5681) -> (1.9183, 15.9288)
  line L162 (1.9183, 15.9288) -> (3.8251, 15.9288)
  line L163 (-0.7073, 15.9288) -> (-0.2529, 15.9288)
  line L164 (-0.2529, 15.9288) -> (1.0958, 13.3007)
  line L165 (1.0958, 13.3007) -> (1.0958, 15.9288)
  line L166 (1.0958, 15.9288) -> (1.4737, 15.9288)
  line L167 (1.4737, 15.9288) -> (1.4737, 12.8808)
  line L168 (1.4737, 12.8808) -> (0.8982, 12.8808)
  line L169 (0.8982, 12.8808) -> (-0.3294, 15.294)
  line L170 (-0.3294, 15.294) -> (-0.3294, 12.8808)
  line L171 (-0.3294, 12.8808) -> (-0.7073, 12.8808)
  line L172 (-0.7073, 12.8808) -> (-0.7073, 15.9288)
  spline S153 degree 2 poles (-2.6018, 15.988) (-2.2783, 15.988) (-1.7423, 15.7904) (-1.5496, 15.5904) knots 0 0 0 1 2 2 2
  spline S154 degree 2 poles (-1.5496, 15.5904) (-1.3569, 15.3878) (-1.1519, 14.7901) (-1.1519, 14.4023) knots 0 0 0 1 2 2 2
  spline S155 degree 2 poles (-1.1519, 14.4023) (-1.1519, 14.0343) (-1.3594, 13.4513) (-1.5521, 13.2438) knots 0 0 0 1 2 2 2
  spline S156 degree 2 poles (-1.5521, 13.2438) (-1.7373, 13.0438) (-2.2807, 12.8264) (-2.6043, 12.8264) knots 0 0 0 1 2 2 2
  spline S157 degree 2 poles (-2.6043, 12.8264) (-2.7599, 12.8264) (-3.0415, 12.8709) (-3.1699, 12.9104) knots 0 0 0 1 2 2 2
  spline S158 degree 2 poles (-3.1699, 12.9104) (-3.2737, 12.94) (-3.5256, 13.0487) (-3.6022, 13.0882) knots 0 0 0 1 2 2 2
  line L173 (-3.6022, 13.0882) -> (-3.6022, 13.5773)
  line L174 (-3.6022, 13.5773) -> (-3.5676, 13.5773)
  spline S159 degree 2 poles (-3.5676, 13.5773) (-3.491, 13.5106) (-3.3305, 13.3896) (-3.1823, 13.3204) knots 0 0 0 1 2 2 2
  spline S160 degree 2 poles (-3.1823, 13.3204) (-3.0588, 13.2587) (-2.7402, 13.1772) (-2.5574, 13.1772) knots 0 0 0 1 2 2 2
  spline S161 degree 2 poles (-2.5574, 13.1772) (-2.1177, 13.1772) (-1.5743, 13.8391) (-1.5743, 14.3899) knots 0 0 0 1 2 2 2
  spline S162 degree 2 poles (-1.5743, 14.3899) (-1.5743, 14.6962) (-1.7176, 15.1556) (-1.8534, 15.3137) knots 0 0 0 1 2 2 2
  spline S163 degree 2 poles (-1.8534, 15.3137) (-1.9843, 15.4718) (-2.3548, 15.6373) (-2.587, 15.6373) knots 0 0 0 1 2 2 2
  spline S164 degree 2 poles (-2.587, 15.6373) (-2.7574, 15.6373) (-3.0983, 15.5879) (-3.2144, 15.5385) knots 0 0 0 1 2 2 2
  line L175 (-3.2144, 15.5385) -> (-3.2144, 14.7506)
  line L176 (-3.2144, 14.7506) -> (-2.508, 14.7506)
  line L177 (-2.508, 14.7506) -> (-2.508, 14.3949)
  line L178 (-2.508, 14.3949) -> (-3.6145, 14.3949)
  line L179 (-3.6145, 14.3949) -> (-3.6145, 15.7262)
  spline S165 degree 2 poles (-3.6145, 15.7262) (-3.538, 15.7608) (-3.2762, 15.867) (-3.165, 15.8991) knots 0 0 0 1 2 2 2
  spline S166 degree 2 poles (-3.165, 15.8991) (-3.0143, 15.9436) (-2.7723, 15.988) (-2.6018, 15.988) knots 0 0 0 1 2 2 2
  spline S167 degree 2 poles (-5.4004, 15.988) (-5.0768, 15.988) (-4.5408, 15.7904) (-4.3481, 15.5904) knots 0 0 0 1 2 2 2
  spline S168 degree 2 poles (-4.3481, 15.5904) (-4.1555, 15.3878) (-3.9505, 14.7901) (-3.9505, 14.4023) knots 0 0 0 1 2 2 2
  spline S169 degree 2 poles (-3.9505, 14.4023) (-3.9505, 14.0343) (-4.1579, 13.4513) (-4.3506, 13.2438) knots 0 0 0 1 2 2 2
  spline S170 degree 2 poles (-4.3506, 13.2438) (-4.5359, 13.0438) (-5.0793, 12.8264) (-5.4028, 12.8264) knots 0 0 0 1 2 2 2
  spline S171 degree 2 poles (-5.4028, 12.8264) (-5.5584, 12.8264) (-5.84, 12.8709) (-5.9685, 12.9104) knots 0 0 0 1 2 2 2
  spline S172 degree 2 poles (-5.9685, 12.9104) (-6.0722, 12.94) (-6.3242, 13.0487) (-6.4007, 13.0882) knots 0 0 0 1 2 2 2
  line L180 (-6.4007, 13.0882) -> (-6.4007, 13.5773)
  line L181 (-6.4007, 13.5773) -> (-6.3661, 13.5773)
  spline S173 degree 2 poles (-6.3661, 13.5773) (-6.2896, 13.5106) (-6.129, 13.3896) (-5.9808, 13.3204) knots 0 0 0 1 2 2 2
  spline S174 degree 2 poles (-5.9808, 13.3204) (-5.8573, 13.2587) (-5.5387, 13.1772) (-5.3559, 13.1772) knots 0 0 0 1 2 2 2
  spline S175 degree 2 poles (-5.3559, 13.1772) (-4.9162, 13.1772) (-4.3728, 13.8391) (-4.3728, 14.3899) knots 0 0 0 1 2 2 2
  spline S176 degree 2 poles (-4.3728, 14.3899) (-4.3728, 14.6962) (-4.5161, 15.1556) (-4.652, 15.3137) knots 0 0 0 1 2 2 2
  spline S177 degree 2 poles (-4.652, 15.3137) (-4.7829, 15.4718) (-5.1534, 15.6373) (-5.3855, 15.6373) knots 0 0 0 1 2 2 2
  spline S178 degree 2 poles (-5.3855, 15.6373) (-5.556, 15.6373) (-5.8968, 15.5879) (-6.0129, 15.5385) knots 0 0 0 1 2 2 2
  line L182 (-6.0129, 15.5385) -> (-6.0129, 14.7506)
  line L183 (-6.0129, 14.7506) -> (-5.3065, 14.7506)
  line L184 (-5.3065, 14.7506) -> (-5.3065, 14.3949)
  line L185 (-5.3065, 14.3949) -> (-6.4131, 14.3949)
  line L186 (-6.4131, 14.3949) -> (-6.4131, 15.7262)
  spline S179 degree 2 poles (-6.4131, 15.7262) (-6.3365, 15.7608) (-6.0747, 15.867) (-5.9635, 15.8991) knots 0 0 0 1 2 2 2
  spline S180 degree 2 poles (-5.9635, 15.8991) (-5.8129, 15.9436) (-5.5708, 15.988) (-5.4004, 15.988) knots 0 0 0 1 2 2 2
  line L187 (-9.8711, 15.9288) -> (-8.3841, 15.9288)
  line L188 (-8.3841, 15.9288) -> (-8.3841, 15.6175)
  line L189 (-8.3841, 15.6175) -> (-8.9374, 15.6175)
  line L190 (-8.9374, 15.6175) -> (-8.9374, 13.5748)
  line L191 (-8.9374, 13.5748) -> (-8.3841, 13.5748)
  line L192 (-8.3841, 13.5748) -> (-8.3841, 13.2957)
  spline S181 degree 2 poles (-8.3841, 13.2957) (-8.6978, 13.2957) (-8.9942, 13.1179) (-9.014, 12.8709) knots 0 0 0 1 2 2 2
  line L193 (-9.014, 12.8709) -> (-9.3302, 12.8709)
  line L194 (-9.3302, 12.8709) -> (-9.3302, 15.6175)
  line L195 (-9.3302, 15.6175) -> (-9.8711, 15.6175)
  line L196 (-9.8711, 15.6175) -> (-9.8711, 15.9288)
  spline S182 degree 2 poles (-12.3584, 14.9407) (-12.3584, 15.1754) (-12.2028, 15.5731) (-12.0719, 15.7065) knots 0 0 0 1 2 2 2
  spline S183 degree 2 poles (-12.0719, 15.7065) (-11.936, 15.8472) (-11.5952, 15.993) (-11.3902, 15.993) knots 0 0 0 1 2 2 2
  spline S184 degree 2 poles (-11.3902, 15.993) (-11.1851, 15.993) (-10.8468, 15.8547) (-10.7183, 15.7163) knots 0 0 0 1 2 2 2
  spline S185 degree 2 poles (-10.7183, 15.7163) (-10.5602, 15.5508) (-10.3824, 14.9951) (-10.3824, 14.59) knots 0 0 0 1 2 2 2
  spline S186 degree 2 poles (-10.3824, 14.59) (-10.3824, 14.1923) (-10.5454, 13.5526) (-10.7158, 13.3155) knots 0 0 0 1 2 2 2
  spline S187 degree 2 poles (-10.7158, 13.3155) (-10.8813, 13.0833) (-11.405, 12.8239) (-11.7483, 12.8239) knots 0 0 0 1 2 2 2
  spline S188 degree 2 poles (-11.7483, 12.8239) (-11.8496, 12.8239) (-12.0274, 12.8437) (-12.0941, 12.8659) knots 0 0 0 1 2 2 2
  line L197 (-12.0941, 12.8659) -> (-12.0941, 13.2587)
  line L198 (-12.0941, 13.2587) -> (-12.0768, 13.2587)
  spline S189 degree 2 poles (-12.0768, 13.2587) (-12.02, 13.229) (-11.8125, 13.1772) (-11.694, 13.1772) knots 0 0 0 1 2 2 2
  spline S190 degree 2 poles (-11.694, 13.1772) (-11.3136, 13.1772) (-10.8468, 13.6909) (-10.8023, 14.1948) knots 0 0 0 1 2 2 2
  spline S191 degree 2 poles (-10.8023, 14.1948) (-10.948, 14.0935) (-11.2543, 13.9824) (-11.4371, 13.9824) knots 0 0 0 1 2 2 2
  spline S192 degree 2 poles (-11.4371, 13.9824) (-11.6149, 13.9824) (-11.8817, 14.054) (-12.0274, 14.1627) knots 0 0 0 1 2 2 2
  spline S193 degree 2 poles (-12.0274, 14.1627) (-12.1954, 14.2887) (-12.3584, 14.6789) (-12.3584, 14.9407) knots 0 0 0 1 2 2 2
  spline S194 degree 2 poles (-11.9434, 14.958) (-11.9434, 14.7703) (-11.8446, 14.5159) (-11.736, 14.427) knots 0 0 0 1 2 2 2
  spline S195 degree 2 poles (-11.736, 14.427) (-11.6544, 14.3628) (-11.4519, 14.3208) (-11.3457, 14.3208) knots 0 0 0 1 2 2 2
  spline S196 degree 2 poles (-11.3457, 14.3208) (-11.2024, 14.3208) (-10.9332, 14.4072) (-10.8023, 14.4887) knots 0 0 0 1 2 2 2
  spline S197 degree 2 poles (-10.8023, 14.4887) (-10.7998, 14.5332) (-10.7949, 14.6172) (-10.7949, 14.6814) knots 0 0 0 1 2 2 2
  spline S198 degree 2 poles (-10.7949, 14.6814) (-10.7949, 14.9976) (-10.9184, 15.3854) (-11.0122, 15.4866) knots 0 0 0 1 2 2 2
  spline S199 degree 2 poles (-11.0122, 15.4866) (-11.0987, 15.583) (-11.2864, 15.6595) (-11.3926, 15.6595) knots 0 0 0 1 2 2 2
  spline S200 degree 2 poles (-11.3926, 15.6595) (-11.6396, 15.6595) (-11.9434, 15.3088) (-11.9434, 14.958) knots 0 0 0 1 2 2 2
  spline S201 degree 2 poles (-14.616, 14.4048) (-14.616, 15.2248) (-14.1393, 15.993) (-13.6428, 15.993) knots 0 0 0 1 2 2 2
  spline S202 degree 2 poles (-13.6428, 15.993) (-13.1389, 15.993) (-12.6672, 15.21) (-12.6672, 14.4072) knots 0 0 0 1 2 2 2
  spline S203 degree 2 poles (-12.6672, 14.4072) (-12.6672, 13.5822) (-13.1439, 12.819) (-13.6428, 12.819) knots 0 0 0 1 2 2 2
  spline S204 degree 2 poles (-13.6428, 12.819) (-14.1442, 12.819) (-14.616, 13.6094) (-14.616, 14.4048) knots 0 0 0 1 2 2 2
  spline S205 degree 2 poles (-14.0924, 15.3335) (-14.1516, 15.1828) (-14.201, 14.7184) (-14.201, 14.4048) knots 0 0 0 1 2 2 2
  spline S206 degree 2 poles (-14.201, 14.4048) (-14.201, 14.0911) (-14.1516, 13.6292) (-14.0899, 13.4736) knots 0 0 0 1 2 2 2
  spline S207 degree 2 poles (-14.0899, 13.4736) (-14.0281, 13.3179) (-13.8132, 13.1574) (-13.6428, 13.1574) knots 0 0 0 1 2 2 2
  spline S208 degree 2 poles (-13.6428, 13.1574) (-13.4724, 13.1574) (-13.2525, 13.3179) (-13.1883, 13.4785) knots 0 0 0 1 2 2 2
  spline S209 degree 2 poles (-13.1883, 13.4785) (-13.1266, 13.6341) (-13.0821, 14.1084) (-13.0821, 14.4072) knots 0 0 0 1 2 2 2
  spline S210 degree 2 poles (-13.0821, 14.4072) (-13.0821, 14.7283) (-13.1216, 15.1581) (-13.1859, 15.3261) knots 0 0 0 1 2 2 2
  spline S211 degree 2 poles (-13.1859, 15.3261) (-13.2451, 15.4842) (-13.465, 15.6546) (-13.6428, 15.6546) knots 0 0 0 1 2 2 2
  spline S212 degree 2 poles (-13.6428, 15.6546) (-13.8108, 15.6546) (-14.0306, 15.494) (-14.0924, 15.3335) knots 0 0 0 1 2 2 2
  spline S213 degree 2 poles (-16.1696, 14.758) (-16.1696, 15.3903) (-15.7646, 16.3487) (-15.4064, 16.771) knots 0 0 0 1 2 2 2
  line L199 (-15.4064, 16.771) -> (-14.9371, 16.771)
  line L200 (-14.9371, 16.771) -> (-14.9371, 16.7513)
  spline S214 degree 2 poles (-14.9371, 16.7513) (-15.0952, 16.6105) (-15.4138, 16.198) (-15.5324, 15.951) knots 0 0 0 1 2 2 2
  spline S215 degree 2 poles (-15.5324, 15.951) (-15.6608, 15.6867) (-15.809, 15.0988) (-15.809, 14.758) knots 0 0 0 1 2 2 2
  spline S216 degree 2 poles (-15.809, 14.758) (-15.809, 14.4196) (-15.6583, 13.8194) (-15.5324, 13.5649) knots 0 0 0 1 2 2 2
  spline S217 degree 2 poles (-15.5324, 13.5649) (-15.4089, 13.3105) (-15.0927, 12.9055) (-14.9371, 12.7647) knots 0 0 0 1 2 2 2
  line L201 (-14.9371, 12.7647) -> (-14.9371, 12.7449)
  line L202 (-14.9371, 12.7449) -> (-15.4064, 12.7449)
  spline S218 degree 2 poles (-15.4064, 12.7449) (-15.7621, 13.1673) (-16.1696, 14.1207) (-16.1696, 14.758) knots 0 0 0 1 2 2 2
  point P0 (0, 0)
  constraints: 2 other
emboss "Emboss2" sketch "Sketch10" operation cut depth 1 direction (0, 1, 0)
sketch "Sketch11" plane through (35, -5, 0) normal (0, 0, -1) x (-1, 0, 0)
  line L0 (35, 10) -> (65, 10) projected
  line L1 (65, 10) -> (0, 10)
  line L2 (0, 10) -> (0, 0)
  line L3 (0, 0) -> (65, 0)
  line L4 (65, 0) -> (65, 10)
  point P0 (35, 5)
  constraints: 8 end point, 2 parallel, 1 horizontal, 1 perpendicular
extrude "Extrusion7" add sketch "Sketch11" along normal blind 2
body "Solid1"
